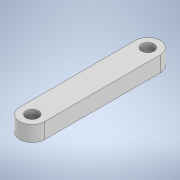
# Autodesk Inventor part: Bar
Saved by Autodesk Inventor 2022 (Build 260153000, 153)
## iProperties
Created: 2021-12-27
Part Number: Bar
Material: Generic
Document SubType Name: Modeling
Designer: kylem
Density: 1 g/cm^3
Appearance: Default
Author: kylem
Autodesk Inventor part; units mm, degrees
ref_plane "YZ Plane" through (0, 0, 0) normal (1, 0, 0) x (0, 1, 0)
ref_plane "XZ Plane" through (0, 0, 0) normal (0, 1, 0) x (-1, 0, 0)
ref_plane "XY Plane" through (0, 0, 0) normal (0, 0, 1) x (1, 0, 0)
sketch "Sketch1" plane through (0, 0, 0) normal (0, 1, 0) x (-1, 0, 0)
  line L0 (0, 0) -> (8, 0)
  line L1 (8, 0) -> (8, -45)
  line L2 (8, -45) -> (0, -45)
  line L3 (0, -45) -> (0, 0)
  line L4 (8, 0) -> (4, 0)
  line L5 (4, 0) -> (4, -4)
  circle A0 centre (4, -4) radius 2
  line L6 (8, -45) -> (4, -45)
  line L7 (4, -45) -> (4, -41)
  circle A1 centre (4, -41) radius 2
  dimension "d0" = 8
  dimension "d1" = 45
  dimension "d2" = 4
  dimension "d3" = 4
  dimension "d4" = 4
  dimension "d5" = 4
  dimension "d6" = 4
  dimension "d7" = 4
  constraints: 16 end point, 3 perpendicular, 2 centre point, 2 coincident, 2 midpoint, 2 parallel, 1 horizontal
  measures "d0" distance of L1.end L2.end
  measures "d1" distance of L0.end L1.end
  measures "d2" distance of L0.end L4.end
  measures "d3" distance of L4.end L5.end
  measures "d4" diameter of A0
  measures "d5" distance of L1.end L6.end
  measures "d6" distance of L6.end L7.end
  measures "d7" diameter of A1
extrude "Extrusion1" add sketch "Sketch1" along normal blind 5
fillet "Fillet1" radius 4 4 edges at (0, 2.5, 0) (-8, 2.5, 0) (-8, 2.5, -45) (0, 2.5, -45)
body "Solid1"
